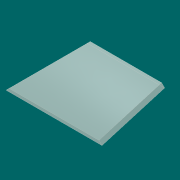
# Autodesk Inventor part: mirrorTopBottom
Saved by Autodesk Inventor 2016 (Build 200138000, 138)
## iProperties
Created: 2015-10-14
Part Number: mirrorTopBottom
Material: Glass
Document SubType Name: Modeling
Designer: Sawaiz
Density: 2.18 g/cm^3
Appearance: Clear
Author: Sawaiz
Autodesk Inventor part; units mm, degrees
ref_plane "XZ Plane" through (0, 0, 0) normal (0, 1, 0) x (-1, 0, 0)
ref_plane "XY Plane" through (0, 0, 0) normal (0, 0, 1) x (1, 0, 0)
sketch "Sketch5" plane through (0, 0, 0) normal (1, 0, 0) x (0, 1, 0)
  line L0 (-50.8, -50.8) -> (50.8, -50.8)
  line L1 (50.8, -50.8) -> (50.8, 50.8)
  line L2 (50.8, 50.8) -> (-50.8, 50.8)
  line L3 (-50.8, 50.8) -> (-50.8, -50.8)
  line L4 (-50.8, -50.8) -> (50.8, 50.8) construction
  line L5 (50.8, -50.8) -> (-50.8, 50.8) construction
  line L6 (-47.625, -47.625) -> (47.625, -47.625)
  line L7 (47.625, -47.625) -> (47.625, 47.625)
  line L8 (47.625, 47.625) -> (-47.625, 47.625)
  line L9 (-47.625, 47.625) -> (-47.625, -47.625)
  line L10 (-47.625, -47.625) -> (47.625, 47.625) construction
  line L11 (47.625, -47.625) -> (-47.625, 47.625) construction
  point P0 (0, 0)
  dimension "d15" = 101.6
  dimension "d16" = 101.6
  dimension "d17" = 95.25
  dimension "d18" = 95.25
  constraints: 24 end point, 4 midpoint, 4 parallel, 2 horizontal, 2 perpendicular
  measures "d15" distance of L2.end L1.end
  measures "d16" distance of L1.end L0.end
  measures "d17" distance of L8.end L7.end
  measures "d18" distance of L7.end L6.end
ref_plane "Work Plane1" through (-76.2, 0, 0) normal (1, 0, 0) x (0, 1, 0)
sketch "Sketch7" plane through (0, 0, 0) normal (0, 1, 0) x (-1, 0, 0)
  line L0 (0, -47.625) -> (76.2, -40.9584)
  line L1 (76.2, -40.9584) -> (76.2, -47.625)
  line L2 (76.2, -47.625) -> (0, -47.625)
  line L3 (0, 47.625) -> (76.2, 47.625)
  line L4 (76.2, 47.625) -> (76.2, 40.9584)
  line L5 (76.2, 40.9584) -> (0, 47.625)
  point P0 (0, 0)
  point P1 (0, 47.625)
  dimension "d21" = 5
  dimension "d22" = 5
  dimension "d23" = 76.2
  constraints: 12 end point, 2 point on line, 1 horizontal, 1 perpendicular, 1 vertical
  measures "d21" angle of L3 L5
  measures "d22" angle of L2 L0
  measures "d23" distance from line of L0.start L1
sketch "Sketch6" plane through (-76.2, 0, 0) normal (1, 0, 0) x (0, 1, 0)
  line L0 (-37.7834, -37.7834) -> (37.7834, -37.7834)
  line L1 (37.7834, -37.7834) -> (37.7834, 37.7834)
  line L2 (37.7834, 37.7834) -> (-37.7834, 37.7834)
  line L3 (-37.7834, 37.7834) -> (-37.7834, -37.7834)
  line L4 (-37.7834, -37.7834) -> (37.7834, 37.7834) construction
  line L5 (37.7834, -37.7834) -> (-37.7834, 37.7834) construction
  line L6 (-40.9584, 40.9584) -> (40.9584, 40.9584)
  line L7 (40.9584, 40.9584) -> (40.9584, -40.9584)
  line L8 (40.9584, -40.9584) -> (-40.9584, -40.9584)
  line L9 (-40.9584, -40.9584) -> (-40.9584, 40.9584)
  point P0 (0, 0)
  point P1 (0, 40.9584)
  point P2 (0, -40.9584)
  dimension "d20" = 3.175
  constraints: 20 end point, 4 parallel, 3 midpoint, 3 perpendicular, 1 horizontal, 3 other
  measures "d20" distance between parallel lines of L2 L6
loft "Loft1" add profiles "Sketch5", "Sketch6" contours L3 L2 L1 L0 | L9 L8 L7 L6 / L3 L2 L1 L0 | L6 L7 L8 L9
sketch "Sketch8" plane through (0, -50.8, -50.8) normal (1, 0, 0) x (0, 0, -1)
  line L0 (0, 0) -> (0, 101.6) projected
  line L1 (0, 101.6) -> (-101.6, 101.6) projected
  line L2 (-101.6, 101.6) -> (-101.6, 0) projected
  line L3 (-101.6, 0) -> (0, 0) projected
  line L4 (-98.425, 3.175) -> (-98.425, 98.425)
  line L5 (-98.425, 98.425) -> (-3.175, 98.425)
  line L6 (-3.175, 98.425) -> (-3.175, 3.175)
  line L7 (-3.175, 3.175) -> (-98.425, 3.175)
  point P0 (-50.8, 50.8)
  dimension "d28" = 3.175
  constraints: 8 end point, 3 other
  measures "d28" distance between parallel lines of L2 L4
sketch "Sketch9" plane through (-76.2, -40.9584, -40.9584) normal (-1, 0, 0) x (0, 0, 1)
  line L0 (0, 0) -> (0, 81.9167) projected
  line L1 (81.9167, 0) -> (0, 0) projected
  line L2 (81.9167, 81.9167) -> (81.9167, 0) projected
  line L3 (0, 81.9167) -> (81.9167, 81.9167) projected
  line L4 (78.7417, 3.175) -> (3.175, 3.175)
  line L5 (3.175, 3.175) -> (3.175, 78.7417)
  line L6 (3.175, 78.7417) -> (78.7417, 78.7417)
  line L7 (78.7417, 78.7417) -> (78.7417, 3.175)
  point P0 (40.9584, 40.9584)
  dimension "d29" = 3.175
  constraints: 8 end point, 3 other
  measures "d29" distance between parallel lines of L2 L7
loft "Loft2" cut profiles "Sketch9", "Sketch8" contours L4 L5 L6 L7 / L4 L5 L6 L7
sketch "Sketch10" plane through (0, -50.8, -50.8) normal (1, 0, 0) x (0, 0, -1)
  line L0 (-3.175, 3.175) -> (-98.425, 3.175) projected
  line L1 (-98.425, 3.175) -> (-98.425, 98.425) projected
  line L2 (-98.425, 98.425) -> (-3.175, 98.425) projected
  line L3 (-3.175, 98.425) -> (-3.175, 3.175) projected
  line L4 (0, 0) -> (0, 101.6) projected
  line L5 (0, 101.6) -> (-101.6, 101.6) projected
  line L6 (-101.6, 101.6) -> (-101.6, 0) projected
  line L7 (-101.6, 0) -> (0, 0) projected
  line L8 (0, 0) -> (-50.8, 50.8)
  line L9 (-50.8, 50.8) -> (0, 101.6)
  constraints: 4 end point, 1 perpendicular
extrude "Extrusion4" cut sketch "Sketch10" against normal through all contours L8 L7 L6 L5 L9 L2 L1 L0 | L0 L1 L2 L9 L8
equation "\"d15\" = width"
equation "\"d16\" = height"
equation "\"d17\" = width - 2 * mirrorThickness"
equation "\"d18\" = height - 2 * mirrorThickness"
equation "\"d21\" = mirrorAngle"
equation "\"d22\" = mirrorAngle"
equation "\"d23\" = focalLength"
equation "\"d20\" = mirrorThickness"
equation "\"d28\" = mirrorThickness"
equation "\"d29\" = mirrorThickness"
equation "\"width\" = 101.6"
equation "\"depth\" = 152.4"
equation "\"mirrorAngle\" = 5deg"
equation "\"mirrorThickness\" = 3.175"
equation "\"fresnelThickness\" = 0.1"
equation "\"centerThickness\" = 1.524"
equation "\"acrylicThickness\" = 6.35"
equation "\"height\" = 101.6"
equation "\"detectorWidth\" = 52"
equation "\"detectorHeight\" = 52"
equation "\"focalLength\" = 76.2"
equation "\"ior\" = 1.49"
equation "\"fresnelAngle\" = 90deg"
equation "\"fresnelEffectiveDiameter\" = 76.2"
equation "\"mirrorSuppourtWidth\" = 38.1"
equation "\"backGrooveBit\" = 4.8006"
equation "\"sensorHolderWidth\" = 88.9"
equation "\"sensorHolderHeight\" = 88.9"
equation "\"sensorHolderSensorHeight\" = 53.975"
equation "\"sensorHolderSensorWidth\" = 53.975"
equation "\"oRingWidth\" = 3.175"
equation "\"sensorHolderORingID\" = 203.2"
equation "\"sensorHolderFlushORingID\" = 304.8"
equation "\"frontBackORingID\" = 419.1"
equation "\"mirrorGroove\" = 19.05"
equation "\"backMirrorGroove\" = 6.35"
equation "\"fresnelMirrorChamfer\" = 6.35"
equation "\"mirrorGrooveMill\" = 3.175"
equation "\"detectorOpeningWidth\" = 76.2"
equation "\"detectorOpeningHeight\" = 76.2"
equation "\"d19\" = -focalLength"
body "Solid2"
